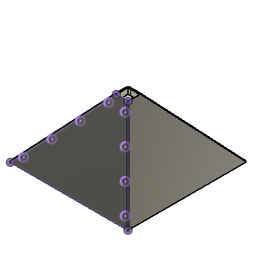
ball_drop_hopper (Autodesk Fusion 360 design; units mm, degrees)
Autodesk Fusion 360 part; units mm, degrees
sketch "Sketch2" plane through (0, 0, 0) normal (0, 0, 1) x (1, 0, 0)
  line L0 (254, -254) -> (-254, -254)
  line L1 (-254, -254) -> (-254, 254)
  line L2 (-254, 254) -> (254, 254)
  line L3 (254, 254) -> (254, -254)
  line L4 (254, -254) -> (-254, 254) construction
  line L5 (-254, -254) -> (254, 254) construction
  dimension "d44" = 508
  dimension "d45" = 508
  constraint horizontal L0
  constraint perpendicular L0 L1
  constraint parallel L0 L2
  constraint parallel L1 L3
  constraint coincident L4 origin
  constraint coincident L5 origin
  measures "d44" distance of L1.end L2.end
  measures "d45" distance of L0.end L1.end
ref_plane "WorkPlane1" through (0, 0, 254) normal (0, 0, 1) x (1, 0, 0)
sketch "Sketch3" plane through (0, 0, 254) normal (0, 0, 1) x (1, 0, 0)
  line L0 (25.4, -25.4) -> (-25.4, -25.4)
  line L1 (-25.4, -25.4) -> (-25.4, 25.4)
  line L2 (-25.4, 25.4) -> (25.4, 25.4)
  line L3 (25.4, 25.4) -> (25.4, -25.4)
  line L4 (25.4, -25.4) -> (-25.4, 25.4) construction
  line L5 (-25.4, -25.4) -> (25.4, 25.4) construction
  dimension "d47" = 50.8
  dimension "d48" = 50.8
  constraint horizontal L0
  constraint perpendicular L0 L1
  constraint parallel L0 L2
  constraint parallel L1 L3
  constraint coincident L4 origin
  constraint coincident L5 origin
  measures "d47" distance of L0.end L1.end
  measures "d48" distance of L1 L3
ref_plane "WorkPlane2" through (-25.4, -25.4, 254) normal (0, -0.743294, 0.668965) x (1, 0, 0)
sketch "Sketch4" plane through (-25.4, -25.4, 254) normal (0, -0.743294, 0.668965) x (1, 0, 0)
  line L0 (50.8, 0) -> (0, 0)
  line L1 (279.4, -341.7221) -> (-228.6, -341.7221)
  line L2 (50.8, 0) -> (279.4, -341.7221)
  line L3 (0, 0) -> (-228.6, -341.7221)
  line L4 (-216.5687, -341.7221) -> (12.0313, 0)
  circle A0 centre (-194.3279, -308.4753) radius 1.7
  circle A1 centre (-10.2096, -33.2467) radius 1.7
  line L5 (-194.3279, -308.4753) -> (-10.2096, -33.2467) construction
  circle A2 centre (-132.9551, -216.7325) radius 1.7
  circle A3 centre (-71.5824, -124.9896) radius 1.7
  line L6 (25.4, -341.7221) -> (25.4, 0) construction
  circle A4 centre (245.1279, -308.4753) radius 1.7
  circle A5 centre (183.7551, -216.7325) radius 1.7
  circle A6 centre (122.3824, -124.9896) radius 1.7
  circle A7 centre (61.0096, -33.2467) radius 1.7
  point P0 (-132.9551, -216.7325)
  point P1 (-71.5824, -124.9896)
  point P2 (-10.2096, -33.2467)
  dimension "d54" = 10
  dimension "d55" = 3.4
  dimension "d56" = 40
  dimension "d57" = 3.4
  dimension "d58" = 40
  dimension "d63" = 331.1349
  dimension "d64" = 0
  dimension "d65" = 3.4
  dimension "d66" = 3.4
  constraint coincident L0.start L2.start
  constraint coincident L1.start L2.end
  constraint coincident L0.end L3.start
  constraint coincident L1.end L3.end
  constraint coincident L1 L4.start
  constraint coincident L0 L4.end
  constraint parallel L3 L4
  constraint coincident L4 A0.centre
  constraint coincident L4 P2
  constraint coincident A0.centre L5.start
  constraint coincident P2 A1.centre
  constraint coincident P0 A2.centre
  constraint coincident P1 A3.centre
  constraint midpoint L1 L6.start
  constraint midpoint L0 L6.end
  constraint symmetric A0 L6 A4
  constraint symmetric A1 L6 A7
  constraint symmetric A2 L6 A5
  constraint symmetric A3 L6 A6
  measures "d54" distance of L3 L4
  measures "d55" diameter of A0
  measures "d56" distance of L4.start A0.centre
  measures "d57" diameter of A1
  measures "d58" distance of L4.end P2
  measures "d65" diameter of A2
  measures "d66" diameter of A3
extrude "Extrude2" add sketch "Sketch4" along normal blind 4.3 contours L0 L1 L2 L4 A0 A1 A2 A3 | L0 L1 L3 L4 A0 A1 A2 A3 makes body 1
ref_plane "WorkPlane3" through (-254, -254, 0) normal (0.743294, 0, -0.668965) x (0, 1, 0)
sketch "Sketch5" plane through (-254, -254, 0) normal (0.743294, 0, -0.668965) x (0, 1, 0)
  line L0 (0, 0) -> (508, 0)
  line L1 (228.6, 341.7221) -> (279.4, 341.7221)
  line L2 (0, 0) -> (228.6, 341.7221)
  line L3 (508, 0) -> (279.4, 341.7221)
  constraint coincident L0.start L2.start
  constraint coincident L1.start L2.end
  constraint coincident L0.end L3.start
  constraint coincident L1.end L3.end
extrude "Extrude3" add sketch "Sketch5" against normal blind 4.3 separate body makes body 2
copy_body "CopyPasteBodies1" bodies 1 2 makes body 3 makes body 4
move_body "Move1" bodies 3 4 to x (-1, 0, 0) y (0, -1, 0) z (0, 0, 1) at (0, 0, 0)
sketch "Sketch6" plane through (-25.4, -25.4, 254) normal (0, -0.743294, 0.668965) x (1, 0, 0)
  circle A0 centre (-132.9551, -216.7325) radius 1.7
  circle A1 centre (-194.3279, -308.4753) radius 1.7
  circle A2 centre (-10.2096, -33.2467) radius 1.7
  circle A3 centre (-71.5824, -124.9896) radius 1.7
  circle A4 centre (245.1279, -308.4753) radius 1.7
  circle A5 centre (183.7551, -216.7325) radius 1.7
  circle A6 centre (122.3824, -124.9896) radius 1.7
  circle A7 centre (61.0096, -33.2467) radius 1.7
  line L0 (50.8, 0) -> (0, 0)
  line L1 (0, 0) -> (-228.6, -341.7221)
  line L2 (-228.6, -341.7221) -> (279.4, -341.7221)
  line L3 (279.4, -341.7221) -> (50.8, 0)
